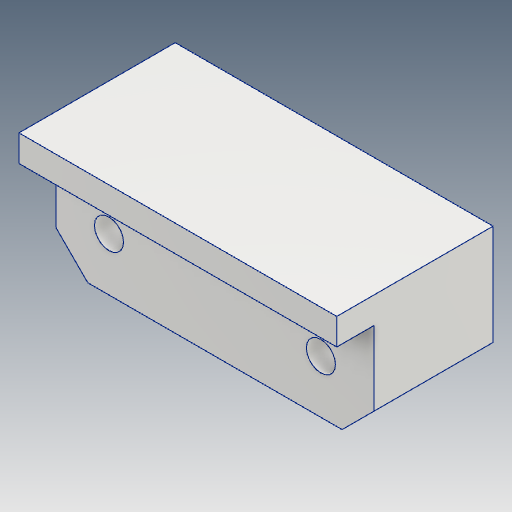
# Autodesk Inventor part: 200-40-BOGIE-CONNECTOR-04
Saved by Autodesk Inventor 2018.2 (Build 222227000, 227)
## iProperties
Manager: feesmrt
Company: FRANC0R
Created: 2017-12-05
Part Number: 200-40-BOGIE-CONNECTOR-04
Material: Aluminium 6061
Document SubType Name: Modeling
Designer: feesmrt
Density: 2.7 g/cm^3
Appearance: Aluminium - flach
Project: Rescue Robot
Cost Center: -
Engineer: feesmrt
Authority: feesmrt
Description: Bogie Connector Part 2
Stock Number: 200-40-BOGIE-CONNECTOR-04
Author: feesmrt
Subject: Rescue Robot
Title: Bogie Connector Part 2
Revision Number: 1
Autodesk Inventor part; units mm, degrees
ref_plane "YZ Plane" through (0, 0, 0) normal (1, 0, 0) x (0, 1, 0)
ref_plane "XZ Plane" through (0, 0, 0) normal (0, 1, 0) x (-1, 0, 0)
ref_plane "XY Plane" through (0, 0, 0) normal (0, 0, 1) x (1, 0, 0)
derived "200-40-BOGIE-CONNECTOR-03.ipt"
sketch "SkizzeAbsatz" plane through (0, 0, 0) normal (0, 1, 0) x (-1, 0, 0)
  line L0 (-30, -74) -> (-30, -55) construction
  line L1 (24, -80) -> (-24, -80) construction
  line L2 (30, -55) -> (30, -74) construction
  line L3 (-30, -55) -> (30, -55) construction
  line L4 (-24, -80) -> (-30, -74) construction
  line L5 (30, -74) -> (24, -80) construction
  circle A0 centre (-20, -70) radius 5 construction
  circle A1 centre (0, -70) radius 2.75 construction
  circle A2 centre (20, -70) radius 5 construction
  circle A3 centre (0, 0) radius 50 construction
  line L6 (0, -106) -> (0, 76) construction
  line L7 (30, 0) -> (30, -74) construction
  line L8 (-30, -74) -> (-30, 0) construction
  line L9 (30, -55) -> (30, -74)
  line L10 (30, -60) -> (-30, -60) construction
  point P0 (0, -50)
sketch "Skizze5" plane through (0, 0, 0) normal (0, 1, 0) x (-1, 0, 0)
  line L0 (-30, -55) -> (30, -55) construction
  line L1 (30, -55) -> (30, -74) construction
  line L2 (30, -74) -> (24, -80) construction
  line L3 (24, -80) -> (-24, -80) construction
  line L4 (-24, -80) -> (-30, -74) construction
  line L5 (-30, -74) -> (-30, -55) construction
  circle A0 centre (-20, -70) radius 5 construction
  circle A1 centre (0, -70) radius 2.75 construction
  circle A2 centre (20, -70) radius 5 construction
  line L6 (30, -55) -> (-30, -55)
  line L7 (-30, -55) -> (-30, -74)
  line L8 (-30, -74) -> (-24, -80)
  line L9 (-24, -80) -> (24, -80)
  line L10 (24, -80) -> (30, -74)
  line L11 (30, -74) -> (30, -55)
  point P0 (0, 0)
  constraints: 12 end point, 2 collinear, 1 horizontal, 1 perpendicular, 1 point on line
extrude "Grundkörper" add sketch "Skizze5" along normal mid plane 22.5
sketch "Skizze7" plane through (0, -11.25, 0) normal (0, -1, 0) x (1, 0, 0)
  line L0 (-30, -60) -> (30, -60) construction
  line L1 (30, -55) -> (-30, -55) projected
  line L2 (30, -74) -> (30, -55) projected
  line L3 (30, -55) -> (-30, -55) projected
  line L4 (-30, -55) -> (-30, -74) projected
  line L5 (-30, -74) -> (-24, -80) projected
  line L6 (-24, -80) -> (24, -80) projected
  line L7 (24, -80) -> (30, -74) projected
  line L8 (30, -74) -> (30, -55) projected
  line L9 (-30, -60) -> (30, -60)
  line L10 (30, -55) -> (30, -74) projected
  point P0 (0, 0)
  dimension "d34" = 5
  constraints: 2 end point, 2 point on line, 1 perpendicular
  measures "d34" distance between parallel lines of L9 L1
extrude "Absatz" add sketch "Skizze7" along normal blind 7 contours L2 L9 L4 L1
sketch "Skizze11" plane through (0, 11.25, 0) normal (0, 1, 0) x (1, 0, 0)
  point P0 (0, 0)
  point P1 (-20, 70)
  point P2 (20, 70)
hole "DIN7984_M5_Boh_T2" at (20, 11.25, -70) at (-20, 11.25, -70) direction (0, -1, 0) diameter 5.5 end through all counterbore diameter 10 counterbore depth 2
sketch "Skizze10" plane through (0, 11.25, 0) normal (0, 1, 0) x (1, 0, 0)
  line L0 (-30, 55) -> (30, 55) projected
  line L1 (30, 55) -> (30, 74) projected
  line L2 (30, 74) -> (24, 80) projected
  line L3 (24, 80) -> (-24, 80) projected
  line L4 (-24, 80) -> (-30, 74) projected
  line L5 (-30, 74) -> (-30, 55) projected
  point P0 (0, 0)
  point P1 (0, 70)
hole "M5x10" at (0, 11.25, -70) direction (0, -1, 0) diameter 4.134 depth 14.2 tip angle 118 countersink diameter 5 countersink angle 90 thread size "M5x0.8" class "6H" standard "ISO Metric profile"
